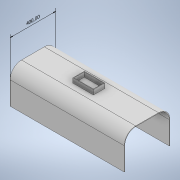
# Autodesk Inventor part: GEAR PANEL
Saved by Autodesk Inventor 2020 (Build 240168000, 168)
## iProperties
Created: 2020-04-01
Part Number: GEAR PANEL
Material: Generic
Document SubType Name: Modeling
Designer: Yusuf
Density: 1 g/cm^3
Appearance: Default
Author: Yusuf
Autodesk Inventor part; units mm, degrees
ref_plane "YZ Plane" through (0, 0, 0) normal (1, 0, 0) x (0, 1, 0)
ref_plane "XZ Plane" through (0, 0, 0) normal (0, 1, 0) x (-1, 0, 0)
ref_plane "XY Plane" through (0, 0, 0) normal (0, 0, 1) x (1, 0, 0)
sketch "Sketch1" plane through (0, 0, 0) normal (0, 1, 0) x (-1, 0, 0)
  line L0 (500, 200) -> (-500, 200)
  line L1 (-500, 200) -> (-500, -200)
  line L2 (-500, -200) -> (500, -200)
  line L3 (500, -200) -> (500, 200)
  line L4 (500, 200) -> (-500, -200) construction
  line L5 (-500, 200) -> (500, -200) construction
  point P0 (0, 0)
  dimension "d0" = 1000
  dimension "d1" = 400
  constraints: 12 end point, 2 midpoint, 2 parallel, 1 horizontal, 1 perpendicular
  measures "d0" distance of L2.end L1.end
  measures "d1" distance of L1.end L0.end
extrude "Extrusion1" add sketch "Sketch1" along normal blind 300
fillet "Fillet1" radius 100 2 edges at (0, 300, 200) (0, 300, -200)
shell "Shell1" thickness 5 removed faces 3 at (-500, 100, -33.3333) at (166.6667, 0, 66.6667) at (500, 100, 33.3333)
sketch "Sketch2" plane through (0, 300, 0) normal (0, 1, 0) x (1, 0, 0)
  line L0 (-100, -50) -> (80, -50)
  line L1 (80, -50) -> (80, 50)
  line L2 (80, 50) -> (-100, 50)
  line L3 (-100, 50) -> (-100, -50)
  line L4 (-500, 100) -> (-500, -100) projected
  line L5 (500, -100) -> (-500, -100) projected
  point P0 (0, 0)
  dimension "d6" = 180
  dimension "d7" = 100
  dimension "d8" = 400
  dimension "d9" = 50
  constraints: 8 end point, 2 parallel, 1 horizontal, 1 perpendicular
  measures "d6" distance of L2.end L1.end
  measures "d7" distance of L1.end L0.end
  measures "d8" distance between parallel lines of L4 L3
  measures "d9" distance between parallel lines of L5 L0
extrude "Extrusion2" add sketch "Sketch2" along normal blind 40
shell "Shell2" thickness 5 removed faces 1 at (-40, 340, 16.6667)
body "Solid1"
